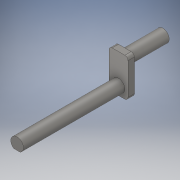
# Autodesk Inventor part: CrankShaft
Saved by Autodesk Inventor 2018 (Build 220112000, 112)
## iProperties
Created: 2017-09-20
Part Number: CrankShaft
Material: Generic
Document SubType Name: Modeling
Designer: Intel
Density: 1 g/cm^3
Appearance: Stainless - Brushed
Author: Intel
Autodesk Inventor part; units mm, degrees
ref_plane "YZ Plane" through (0, 0, 0) normal (1, 0, 0) x (0, 1, 0)
ref_plane "XZ Plane" through (0, 0, 0) normal (0, 1, 0) x (-1, 0, 0)
ref_plane "XY Plane" through (0, 0, 0) normal (0, 0, 1) x (1, 0, 0)
sketch "Sketch1" plane through (0, 0, 0) normal (1, 0, 0) x (0, 1, 0)
  line L0 (-9.525, 36.5125) -> (9.525, 36.5125)
  line L1 (9.525, 36.5125) -> (9.525, -36.5125)
  line L2 (9.525, -36.5125) -> (-9.525, -36.5125)
  line L3 (-9.525, -36.5125) -> (-9.525, 36.5125)
  line L4 (-9.525, 36.5125) -> (9.525, -36.5125) construction
  line L5 (9.525, 36.5125) -> (-9.525, -36.5125) construction
  point P0 (0, 0)
  dimension "d0" = 19.05
  dimension "d1" = 73.025
  constraints: 12 end point, 2 midpoint, 2 parallel, 1 horizontal, 1 perpendicular
  measures "d0" distance of L1.end L2.end
  measures "d1" distance of L0.end L1.end
extrude "Extrusion1" add sketch "Sketch1" along normal mid plane 9.525
sketch "Sketch2" plane through (4.7625, 0, 0) normal (1, 0, 0) x (0, 0, -1)
  line L0 (-36.5125, 9.525) -> (-36.5125, -9.525) projected
  line L1 (-36.5125, 9.525) -> (14.2875, 9.525)
  line L2 (14.2875, 9.525) -> (14.2875, -1.5875)
  line L3 (14.2875, -1.5875) -> (-36.5125, -1.5875)
  line L4 (-36.5125, -1.5875) -> (-36.5125, 9.525)
  line L5 (-36.5125, -9.525) -> (36.5125, -9.525) projected
  point P0 (0, 0)
  dimension "d4" = 50.8
  dimension "d6" = 7.9375
  constraints: 8 end point, 2 parallel, 1 horizontal, 1 perpendicular
  measures "d4" distance of L2.end L3.end
  measures "d6" distance between parallel lines of L5 L3
extrude "Extrusion2" cut sketch "Sketch2" against normal blind 9.525
sketch "Sketch3" plane through (4.7625, 0, 0) normal (1, 0, 0) x (0, 0, -1)
  line L0 (36.5125, -9.525) -> (-36.5125, -9.525) projected
  line L1 (36.5125, -9.525) -> (17.4625, -9.525)
  line L2 (17.4625, -9.525) -> (17.4625, 1.5875)
  line L3 (17.4625, 1.5875) -> (36.5125, 1.5875)
  line L4 (36.5125, 1.5875) -> (36.5125, -9.525)
  line L5 (14.2875, 9.525) -> (14.2875, -1.5875) projected
  line L6 (36.5125, 9.525) -> (14.2875, 9.525) projected
  point P0 (0, 0)
  dimension "d9" = 3.175
  dimension "d10" = 7.9375
  constraints: 8 end point, 2 parallel, 1 horizontal, 1 perpendicular
  measures "d9" distance between parallel lines of L5 L2
  measures "d10" distance between parallel lines of L6 L3
extrude "Extrusion3" cut sketch "Sketch3" against normal blind 9.525
sketch "Sketch4" plane through (4.7625, 0, 0) normal (1, 0, 0) x (0, 0, -1)
  line L0 (-36.5125, -1.5875) -> (-36.5125, -9.525) projected
  line L1 (-36.5125, -9.525) -> (14.2875, -9.525)
  line L2 (14.2875, -9.525) -> (14.2875, -7.9375)
  line L3 (14.2875, -7.9375) -> (-36.5125, -7.9375)
  line L4 (-36.5125, -7.9375) -> (-36.5125, -9.525)
  point P0 (0, 0)
  dimension "d13" = 50.8
  dimension "d14" = 1.5875
  constraints: 8 end point, 2 parallel, 1 horizontal, 1 perpendicular
  measures "d13" distance of L3.end L2.end
  measures "d14" distance of L2.end L1.end
extrude "Extrusion4" cut sketch "Sketch4" against normal blind 9.525
sketch "Sketch5" plane through (4.7625, 0, 0) normal (1, 0, 0) x (0, 0, -1)
  line L0 (36.5125, 9.525) -> (36.5125, 1.5875) projected
  line L1 (36.5125, 9.525) -> (17.4625, 9.525)
  line L2 (17.4625, 9.525) -> (17.4625, 7.9375)
  line L3 (17.4625, 7.9375) -> (36.5125, 7.9375)
  line L4 (36.5125, 7.9375) -> (36.5125, 9.525)
  point P0 (0, 0)
  dimension "d17" = 19.05
  dimension "d18" = 1.5875
  constraints: 8 end point, 2 parallel, 1 horizontal, 1 perpendicular
  measures "d17" distance of L3.end L2.end
  measures "d18" distance of L2.end L1.end
extrude "Extrusion5" cut sketch "Sketch5" against normal blind 9.525
sketch "Sketch7" plane through (4.7625, 1.5875, -36.5125) normal (0, 0, -1) x (-1, 0, 0)
  line L0 (9.525, 6.35) -> (9.525, 0) projected
  line L1 (0, 0) -> (0, 6.35) projected
  line L2 (9.525, 6.35) -> (0, 6.35)
  line L3 (0, 6.35) -> (0, 0)
  line L4 (0, 0) -> (9.525, 0)
  line L5 (9.525, 0) -> (9.525, 6.35)
  circle A0 centre (4.7625, 3.81) radius 3.175
  point P0 (4.7625, -1.5875)
  dimension "d26" = 6.35
  dimension "d27" = 4.7625
  dimension "d28" = 3.81
  constraints: 8 end point, 2 parallel, 1 centre point, 1 horizontal, 1 perpendicular
  measures "d26" diameter of A0
  measures "d27" distance from line of L0 A0.centre
  measures "d28" distance from line of L4 A0.centre
extrude "Extrusion7" add sketch "Sketch7" against normal blind 19.05 contours A0 L2 | L2 A0
sketch "Sketch6" plane through (-4.7625, -1.5875, 36.5125) normal (0, 0, 1) x (1, 0, 0)
  line L0 (9.525, -6.35) -> (0, -6.35) projected
  line L1 (9.525, 0) -> (0, 0) projected
  line L2 (0, -6.35) -> (9.525, -6.35)
  line L3 (9.525, -6.35) -> (9.525, 0)
  line L4 (9.525, 0) -> (0, 0)
  line L5 (0, 0) -> (0, -6.35)
  circle A0 centre (4.7625, -3.6322) radius 3.175
  point P0 (4.7625, 1.5875)
  dimension "d21" = 6.35
  dimension "d22" = 3.6322
  dimension "d23" = 4.7625
  constraints: 8 end point, 2 parallel, 1 centre point, 1 horizontal, 1 perpendicular
  measures "d21" diameter of A0
  measures "d22" distance from line of L1 A0.centre
  measures "d23" distance from line of L3 A0.centre
extrude "Extrusion6" cut sketch "Sketch6" against normal blind 50.8 contours L0 A0 L5 L1 L3
fillet "Fillet1" radius 1.5875 4 edges at (4.7625, 9.525, -15.875) (-4.7625, 9.525, -15.875) (4.7625, -9.525, -15.875) (-4.7625, -9.525, -15.875)
sketch "Sketch8" plane through (4.7625, 1.5875, -36.5125) normal (0, 0, -1) x (-1, 0, 0)
  arc A0 (6.6675, 6.35) -> (2.8575, 6.35) centre (4.7625, 3.81) ccw projected
  circle A1 centre (4.7625, 3.81) radius 3.175
  line L0 (0, 6.35) -> (2.8575, 6.35) projected
  line L1 (2.8575, 6.35) -> (0, 6.35)
  line L2 (0, 0) -> (0, 6.35) projected
  line L3 (0, 0) -> (9.525, 0) projected
  line L4 (9.525, 6.35) -> (9.525, 0) projected
  line L5 (2.8575, 6.35) -> (0, 6.35) projected
  line L6 (0, 0) -> (0, 6.35) projected
  line L7 (0, 0) -> (9.525, 0) projected
  line L8 (9.525, 6.35) -> (9.525, 0) projected
  line L9 (9.525, 6.35) -> (6.6675, 6.35) projected
  arc A2 (6.6675, 6.35) -> (2.8575, 6.35) centre (4.7625, 3.81) ccw projected
  line L10 (0, 0) -> (9.525, 0) projected
  line L11 (0, 6.35) -> (0, 0)
  line L12 (0, 0) -> (9.525, 0)
  line L13 (9.525, 0) -> (9.525, 6.35)
  point P0 (4.7625, -1.5875)
  constraints: 8 end point, 1 centre point, 1 coincident, 1 collinear, 1 horizontal, 1 perpendicular, 1 vertical
extrude "Extrusion8" cut sketch "Sketch8" against normal blind 19.05 contours L9 L4 L3 L2 L0 A1
body "Solid1"
